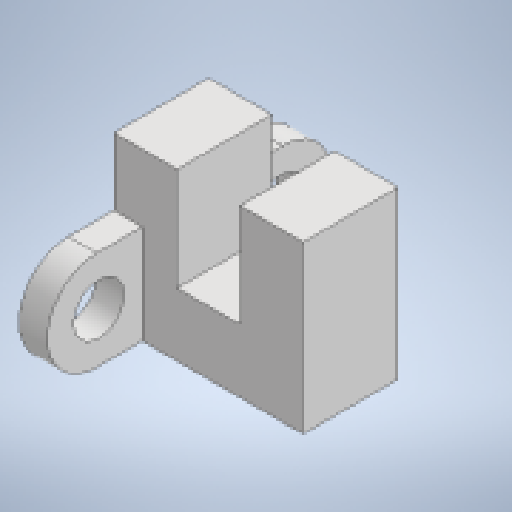
# Autodesk Inventor part: TP806 optic endstop
Saved by Autodesk Inventor 2025 (Build 290162000, 162)
## iProperties
Created: 2025-07-05
Part Number: TP806 optic endstop
Material: 一般
Document SubType Name: Modeling
Designer: gavin
Density: 1 g/cm^3
Appearance: 預設
Author: gavin
Autodesk Inventor part; units mm, degrees
ref_plane "YZ Plane" through (0, 0, 0) normal (1, 0, 0) x (0, 1, 0)
ref_plane "XZ Plane" through (0, 0, 0) normal (0, 1, 0) x (-1, 0, 0)
ref_plane "XY Plane" through (0, 0, 0) normal (0, 0, 1) x (1, 0, 0)
sketch "草圖1" plane through (0, 0, 0) normal (1, 0, 0) x (0, 1, 0)
  line L0 (0, 9) -> (0, 9)
  line L1 (-3.125, 5.875) -> (-3.125, -5.875)
  line L2 (0, -9) -> (0, -9)
  line L3 (3.125, -5.875) -> (3.125, 5.875)
  line L4 (3.125, 9) -> (-3.125, -9) construction
  line L5 (-3.125, 9) -> (3.125, -9) construction
  circle A0 centre (0, 5.75) radius 1.6
  circle A1 centre (0, -5.75) radius 1.6
  arc A2 (0, -9) -> (3.125, -5.875) centre (0, -5.875) ccw
  arc A3 (-3.125, -5.875) -> (0, -9) centre (0, -5.875) ccw
  arc A4 (0, 9) -> (-3.125, 5.875) centre (0, 5.875) ccw
  arc A5 (3.125, 5.875) -> (0, 9) centre (0, 5.875) ccw
  point P0 (0, 0)
  point P1 (0, 0)
  point P2 (0, -9)
  point P3 (0, 9)
  dimension "d2" = 6.25
  dimension "d3" = 18
  dimension "d4" = 3.2
  dimension "d5" = 3.2
  dimension "d6" = 11.5
  dimension "d7" = 5.75
  dimension "d8" = 3.125
  dimension "d9" = 3.125
  constraints: 12 end point, 8 point on circle, 8 point on line, 8 tangent, 6 centre point, 2 equal radius, 2 midpoint, 2 parallel, 1 coincident, 1 horizontal, 1 perpendicular, 1 other
  measures "d2" distance of L4.end L5.end
  measures "d3" distance of L5.start L4.end
  measures "d4" diameter of A0
  measures "d5" diameter of A1
  measures "d6" distance of A1.centre A0.centre
  measures "d7" distance of point (0, 0) A1.centre
  measures "d8" radius of A2
  measures "d9" radius of A3
extrude "擠出1" add sketch "草圖1" along normal blind 1.8
sketch "草圖2" plane through (0, 0, 0) normal (0, 0, 1) x (1, 0, 0)
  line L0 (0, -3.125) -> (0, 3.125) projected
  line L1 (0, -3.125) -> (0, 7.375)
  line L2 (0, 7.375) -> (4, 7.375)
  line L3 (4, 7.375) -> (4, 0.875)
  line L4 (4, 0.875) -> (7.98, 0.875)
  line L5 (7.98, 0.875) -> (7.98, 7.375)
  line L6 (7.98, 7.375) -> (11.98, 7.375)
  line L7 (11.98, 7.375) -> (11.98, -3.125)
  line L8 (11.98, -3.125) -> (0, -3.125)
  point P0 (0, 0)
  dimension "d12" = 10.5
  dimension "d13" = 4
  dimension "d14" = 3.98
  dimension "d15" = 4
  dimension "d16" = 6.5
  constraints: 16 end point, 6 perpendicular, 2 point on line, 1 vertical
  measures "d12" distance of L0.start L1.end
  measures "d13" distance of L1.end L2.end
  measures "d14" distance of L3.end L4.end
  measures "d15" distance of L5.end L6.end
  measures "d16" distance of L4.end L5.end
extrude "擠出2" add sketch "草圖2" along normal mid plane 6
equation "\"d7\" = 0.5 * d6"
